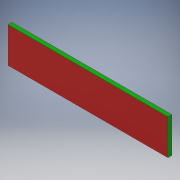
# Autodesk Inventor part: ButtonBoard
Saved by Autodesk Inventor 2019.3 (Build 233278000, 278)
## iProperties
Created: 2019-03-27
Part Number: ButtonBoard
Material: Generic
Document SubType Name: Modeling
Designer: Willist
Density: 1 g/cm^3
Appearance: Default
Author: Willist
Autodesk Inventor part; units mm, degrees
ref_plane "YZ Plane" through (0, 0, 0) normal (1, 0, 0) x (0, 1, 0)
ref_plane "XZ Plane" through (0, 0, 0) normal (0, 1, 0) x (-1, 0, 0)
ref_plane "XY Plane" through (0, 0, 0) normal (0, 0, 1) x (1, 0, 0)
sketch "Sketch1" plane through (0, 0, 0) normal (0, 0, 1) x (1, 0, 0)
  line L0 (45, 10) -> (-45, 10)
  line L1 (-45, 10) -> (-45, -10)
  line L2 (-45, -10) -> (45, -10)
  line L3 (45, -10) -> (45, 10)
  point P0 (0, 0)
  dimension "d0" = 90
  dimension "d1" = 20
  constraints: 8 end point, 2 parallel, 1 horizontal, 1 perpendicular
  measures "d0" distance of L2.end L1.end
  measures "d1" distance of L1.end L0.end
extrude "Extrusion1" add sketch "Sketch1" along normal blind 2.17
body "Solid1"
